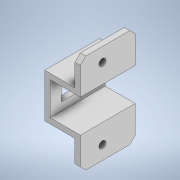
# Autodesk Inventor part: houder motor
Saved by Autodesk Inventor 2022 (Build 260153000, 153)
## iProperties
Created: 2022-10-16
Part Number: houder motor
Material: Generic
Document SubType Name: Modeling
Designer: devol
Density: 1 g/cm^3
Appearance: Default
Author: devol
Autodesk Inventor part; units mm, degrees
ref_plane "YZ Plane" through (0, 0, 0) normal (1, 0, 0) x (0, 1, 0)
ref_plane "XZ Plane" through (0, 0, 0) normal (0, 1, 0) x (-1, 0, 0)
ref_plane "XY Plane" through (0, 0, 0) normal (0, 0, 1) x (1, 0, 0)
sketch "Sketch1" plane through (0, 0, 0) normal (1, 0, 0) x (0, 1, 0)
  line L0 (0, 0) -> (16, 0)
  line L1 (16, 0) -> (16, -24)
  line L2 (16, -24) -> (0, -24)
  line L3 (0, -24) -> (0, 0)
  dimension "d0" = 16
  dimension "d1" = 24
  constraints: 8 end point, 2 parallel, 1 horizontal, 1 perpendicular
  measures "d0" distance of L1.end L2.end
  measures "d1" distance of L0.end L1.end
extrude "Extrusion1" add sketch "Sketch1" along normal blind 2
sketch "Sketch2" plane through (2, 0, 0) normal (1, 0, 0) x (0, 0, -1)
  line L0 (24, 16) -> (0, 16) projected
  line L1 (0, 16) -> (24, 16)
  line L2 (24, 16) -> (24, 14)
  line L3 (24, 14) -> (0, 14)
  line L4 (0, 14) -> (0, 16)
  line L5 (0, 16) -> (0, 0) projected
  line L6 (0, 0) -> (24, 0)
  line L7 (24, 0) -> (24, 2)
  line L8 (24, 2) -> (0, 2)
  line L9 (0, 2) -> (0, 0)
  dimension "d4" = 24
  dimension "d5" = 2
  dimension "d6" = 24
  dimension "d7" = 2
  constraints: 16 end point, 4 parallel, 2 horizontal, 2 perpendicular
  measures "d4" distance of L2.end L3.end
  measures "d5" distance of L1.end L2.end
  measures "d6" distance of L8.end L7.end
  measures "d7" distance of L7.end L6.end
extrude "Extrusion2" add sketch "Sketch2" along normal blind 11
sketch "Sketch3" plane through (0, 0, -24) normal (0, -1, 0) x (1, 0, 0)
  line L0 (13, 24) -> (11, 24)
  line L1 (11, 24) -> (11, 0)
  line L2 (11, 0) -> (13, 0)
  line L3 (13, 0) -> (13, 24)
  point P0 (0, 24)
  dimension "d10" = 2
  dimension "d11" = 24
  constraints: 8 end point, 2 parallel, 1 horizontal, 1 perpendicular
  measures "d10" distance of L2.end L1.end
  measures "d11" distance of L1.end L0.end
extrude "Extrusion3" add sketch "Sketch3" along normal blind 10
sketch "Sketch4" plane through (0, 16, 0) normal (0, 1, 0) x (1, 0, 0)
  line L0 (13, 24) -> (13, 0) projected
  line L1 (13, 24) -> (11, 24)
  line L2 (11, 24) -> (11, 0)
  line L3 (11, 0) -> (13, 0)
  line L4 (13, 0) -> (13, 24)
  point P0 (0, 0)
  point P1 (13, 0)
  dimension "d14" = 2
  dimension "d15" = 24
  constraints: 8 end point, 2 parallel, 1 horizontal, 1 perpendicular
  measures "d14" distance of L3.end L2.end
  measures "d15" distance of L2.end L1.end
extrude "Extrusion4" add sketch "Sketch4" along normal blind 10
sketch "Sketch5" plane through (13, 0, 0) normal (1, 0, 0) x (0, 0, -1)
  line L0 (0, 0) -> (0, -5)
  line L1 (0, 2) -> (0, -10) projected
  line L2 (0, -5) -> (12, -5)
  line L3 (24, 0) -> (24, -10) projected
  circle A0 centre (12, -5) radius 1.25
  line L4 (0, 14) -> (24, 14) projected
  line L5 (0, 14) -> (0, 21)
  line L6 (0, 14) -> (0, 26) projected
  line L7 (0, 21) -> (12, 21)
  circle A1 centre (12, 21) radius 1.25
  dimension "d18" = 5
  dimension "d19" = 12
  dimension "d20" = 2.5
  dimension "d21" = 7
  dimension "d22" = 12
  dimension "d23" = 2.5
  constraints: 8 end point, 2 centre point, 2 coincident, 2 perpendicular, 2 point on line
  measures "d18" distance of L0.start L0.end
  measures "d19" distance of L0.end L2.end
  measures "d20" diameter of A0
  measures "d21" distance of L4.start L5.end
  measures "d22" distance of L5.end L7.end
  measures "d23" diameter of A1
extrude "Extrusion5" cut sketch "Sketch5" against normal blind 10
sketch "Sketch7" plane through (0, 0, 0) normal (-1, 0, 0) x (0, 0, 1)
  line L0 (-20, 5) -> (-8, 5)
  line L1 (-8, 5) -> (-8, 11)
  line L2 (-8, 11) -> (-20, 11)
  line L3 (-20, 11) -> (-20, 5)
  line L4 (-24, 0) -> (-24, 16) projected
  point P0 (0, 0)
  dimension "d26" = 6
  dimension "d27" = 12
  dimension "d28" = 5
  dimension "d29" = 4
  constraints: 8 end point, 2 parallel, 1 horizontal, 1 perpendicular
  measures "d26" distance of L2.end L0.start
  measures "d27" distance between parallel lines of L1 L3
  measures "d28" distance from line of L0 point (0, 0)
  measures "d29" distance between parallel lines of L4 L3
extrude "Extrusion6" cut sketch "Sketch7" against normal blind 10
sketch "Sketch8" plane through (0, 0, 0) normal (0, 0, 1) x (1, 0, 0)
  line L0 (11, -10) -> (13, -10) projected
  line L1 (11, -10) -> (13, -10)
  line L2 (13, 2) -> (13, -10) projected
  line L3 (13, -10) -> (13, 2)
  line L4 (2, 2) -> (13, 2) projected
  line L5 (13, 2) -> (2, 2)
  line L6 (2, 14) -> (2, 2) projected
  line L7 (2, 2) -> (2, 14)
  line L8 (13, 14) -> (13, 26) projected
  line L9 (2, 14) -> (13, 14)
  line L10 (13, 14) -> (13, 26)
  line L11 (11, 16) -> (11, 26) projected
  line L12 (13, 26) -> (11, 26)
  line L13 (11, 26) -> (11, 16)
  line L14 (11, 16) -> (0, 16)
  line L15 (0, 0) -> (11, 0) projected
  line L16 (0, 16) -> (0, 0)
  line L17 (0, 0) -> (11, 0)
  line L18 (11, 0) -> (11, -10) projected
  line L19 (11, 0) -> (11, -10)
  constraints: 24 end point, 8 perpendicular, 4 collinear
extrude "Extrusion7" cut sketch "Sketch8" against normal blind 4
chamfer "Chamfer1" distance 2 angle 45 2 edges at (12, -10, -24) (12, 26, -24)
chamfer "Chamfer2" distance 2 angle 45 2 edges at (12, -10, -4) (12, 26, -4)
body "Solid1"
